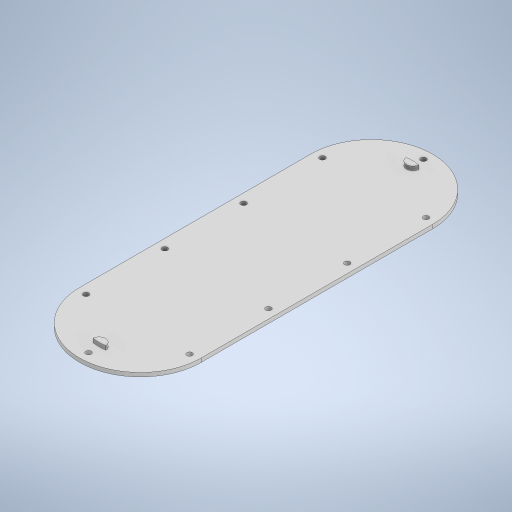
# Autodesk Inventor part: top_housing_base-plate
Saved by Autodesk Inventor 2023.1 (Build 271208000, 208)
## iProperties
Created: 2026-05-20
Part Number: top_housing_base-plate
Material: Generic
Document SubType Name: Modeling
Designer: Lars
Density: 1 g/cm^3
Appearance: Default
Author: Lars
Autodesk Inventor part; units mm, degrees
ref_plane "YZ Plane" through (0, 0, 0) normal (1, 0, 0) x (0, 1, 0)
ref_plane "XZ Plane" through (0, 0, 0) normal (0, 1, 0) x (-1, 0, 0)
ref_plane "XY Plane" through (0, 0, 0) normal (0, 0, 1) x (1, 0, 0)
sketch "Sketch1" plane through (0, 0, 0) normal (0, 1, 0) x (-1, 0, 0)
  line L0 (0, 121.25) -> (0, 121.25)
  line L1 (32, 89.25) -> (32, -89.25)
  line L2 (0, -121.25) -> (0, -121.25)
  line L3 (-32, -89.25) -> (-32, 89.25)
  line L4 (32, 0) -> (-32, 0) construction
  arc A0 (32, 89.25) -> (0, 121.25) centre (0, 89.25) ccw
  arc A1 (0, 121.25) -> (-32, 89.25) centre (0, 89.25) ccw
  arc A2 (0, -121.25) -> (32, -89.25) centre (0, -89.25) ccw
  arc A3 (-32, -89.25) -> (0, -121.25) centre (0, -89.25) ccw
  arc A4 (0, -136.25) -> (47, -89.25) centre (0, -89.25) ccw
  line L5 (47, -89.25) -> (47, 89.25)
  arc A5 (47, 89.25) -> (-34.4238, 121.25) centre (0, 89.25) ccw
  arc A6 (-34.4238, 121.25) -> (-47, 89.25) centre (0, 89.25) ccw
  line L6 (-47, 89.25) -> (-47, -89.25)
  arc A7 (-47, -89.25) -> (0, -136.25) centre (0, -89.25) ccw
  arc A8 (0, 129.25) -> (-40, 89.25) centre (0, 89.25) ccw construction
  line L7 (-40, 89.25) -> (-40, -89.25) construction
  arc A9 (-40, -89.25) -> (24, -121.25) centre (0, -89.25) ccw construction
  arc A10 (24, -121.25) -> (40, -89.25) centre (0, -89.25) ccw construction
  line L8 (40, -89.25) -> (40, 89.25) construction
  arc A11 (40, 89.25) -> (0, 129.25) centre (0, 89.25) ccw construction
  circle A12 centre (0, -129.25) radius 2.05
  circle A13 centre (0, 129.25) radius 2.05
  circle A14 centre (-39.9488, 91.2737) radius 2.05
  circle A15 centre (39.9488, 91.2737) radius 2.05
  circle A16 centre (-40, 30.42) radius 2.05
  circle A17 centre (40, 30.42) radius 2.05
  circle A18 centre (0, -129.25) radius 2.05
  circle A19 centre (-39.9488, -91.2737) radius 2.05
  circle A20 centre (39.9488, -91.2737) radius 2.05
  circle A21 centre (-40, -30.42) radius 2.05
  circle A22 centre (40, -30.42) radius 2.05
  circle A23 centre (0, 121.25) radius 5
  circle A24 centre (0, -121.25) radius 5
  point P0 (0, 0)
  point P1 (32, -121.25)
  point P2 (32, 121.25)
  point P3 (-32, -121.25)
  point P4 (0, 0)
  point P5 (-40, 0)
  point P6 (40, 0)
  point P7 (4.9847, -120.8594)
  point P8 (-4.9847, -120.8594)
  point P9 (0, -121.25)
  point P10 (-4.9847, 120.8594)
  point P11 (4.9847, 120.8594)
  point P12 (0, 121.25)
  dimension "d0" = 242.5
  dimension "d1" = 64
  dimension "d2" = 32
  dimension "d3" = 32
  dimension "d4" = 15
  dimension "d5" = 8
  dimension "d6" = 4.1
  dimension "d7" = 4.1
  dimension "d10" = 87.1
  dimension "d14" = 87.1
  dimension "d16" = 4.1
  dimension "d17" = 30.42
  dimension "d18" = 4.1
  dimension "d19" = 30.42
  dimension "d20" = 10
  dimension "d21" = 10
  constraints: 25 centre point, 25 point on circle, 18 end point, 8 point on line, 8 tangent, 6 coincident, 5 midpoint, 5 symmetric about line, 4 parallel, 2 concentric, 1 horizontal, 1 perpendicular, 23 other
  measures "d0" distance of point (32, 121.25) point (32, -121.25)
  measures "d1" distance of point (32, -121.25) point (-32, -121.25)
  measures "d2" radius of A0
  measures "d3" radius of A2
  measures "d4" radial gap between concentric circles of A3 A7
  measures "d5" radial gap between concentric circles of A0 A11
  measures "d6" diameter of A12
  measures "d7" diameter of A13
  measures "d16" diameter of A16
  measures "d17" distance of point (-40, 0) A16.centre
  measures "d18" diameter of A17
  measures "d19" distance of point (40, 0) A17.centre
  measures "d20" diameter of A23
  measures "d21" diameter of A24
extrude "Extrusion1" add sketch "Sketch1" against normal blind 3 contours L1 A2 A24 A3 L3 A1 A23 A0 | A23 A1 A0 | A0 A1 A23 | A24 A3 A2 | A2 A3 A24 | A7 L6 A6 A5 L5 A4
extrude "Extrusion2" add sketch "Sketch1" along normal blind 3 contours A23 A1 A0 | A2 A3 A24 picked at (0.9662, 119.6201) picked at (0.9662, -119.6201)
body "Solid1"
